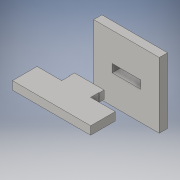
# Autodesk Inventor part: Part1
Saved by Autodesk Inventor 2016 (Build 200138000, 138)
## iProperties
Created: 2017-09-21
Part Number: Part1
Material: Generic
Document SubType Name: Modeling
Designer: student
Density: 1 g/cm^3
Appearance: Default
Author: student
Autodesk Inventor part; units mm, degrees
ref_plane "YZ Plane" through (0, 0, 0) normal (1, 0, 0) x (0, 1, 0)
ref_plane "XZ Plane" through (0, 0, 0) normal (0, 1, 0) x (-1, 0, 0)
ref_plane "XY Plane" through (0, 0, 0) normal (0, 0, 1) x (1, 0, 0)
sketch "Sketch1" plane through (0, 0, 0) normal (0, 0, 1) x (1, 0, 0)
  line L0 (-14.792, -1.3102) -> (-14.792, 1.814)
  line L1 (-14.792, 1.814) -> (-3.743, 1.814)
  line L2 (-3.743, 1.814) -> (-3.743, -1.3102)
  line L3 (-3.743, -1.3102) -> (-14.792, -1.3102)
  line L4 (-21.9675, -12.4544) -> (3.4325, -12.4544)
  line L5 (3.4325, -12.4544) -> (3.4325, 12.9456)
  line L6 (3.4325, 12.9456) -> (-21.9675, 12.9456)
  line L7 (-21.9675, 12.9456) -> (-21.9675, -12.4544)
  line L8 (-21.9675, -12.4544) -> (3.4325, 12.9456) construction
  line L9 (3.4325, -12.4544) -> (-21.9675, 12.9456) construction
  point P0 (0, 0)
  point P1 (-9.2675, 0.2456)
  dimension "d0" = 3.1242
  dimension "d2" = 11.049
  dimension "d3" = 25.4
  dimension "d4" = 25.4
  constraints: 20 end point, 2 horizontal, 2 midpoint, 2 parallel, 2 perpendicular, 2 vertical
  measures "d0" distance of L0.start L0.end
  measures "d2" distance of L0.end L1.end
  measures "d3" distance of L6.end L5.end
  measures "d4" distance of L5.end L4.end
extrude "Extrusion1" add sketch "Sketch1" along normal blind 3.175
sketch "Sketch2" plane through (0, 0, 0) normal (0, 1, 0) x (-1, 0, 0)
  line L0 (17.4601, 16.8923) -> (17.4601, 20.0673)
  line L1 (6.2587, 16.8923) -> (6.2587, 20.0673)
  line L2 (6.2587, 20.0673) -> (-3.2663, 20.0673)
  line L3 (17.4601, 20.0673) -> (26.9851, 20.0673)
  line L4 (26.9851, 20.0673) -> (26.9851, 29.5923)
  line L5 (26.9851, 29.5923) -> (-3.2663, 29.5923)
  line L6 (-3.2663, 29.5923) -> (-3.2663, 20.0673)
  line L7 (17.4601, 16.8923) -> (17.5871, 16.8923)
  line L8 (6.2587, 16.8923) -> (6.1317, 16.8923)
  line L9 (6.1317, 16.8923) -> (6.1317, 14.9873)
  line L10 (6.1317, 14.9873) -> (17.5871, 14.9873)
  line L11 (17.5871, 14.9873) -> (17.5871, 16.8923)
  point P0 (0, 0)
  dimension "d10" = 9.525
  dimension "d11" = 9.525
  dimension "d12" = 9.525
  dimension "d14" = 0.127
  dimension "d15" = 0.127
  dimension "d16" = 1.905
  dimension "d19" = 11.2014
  dimension "d20" = 11.4554
  constraints: 24 end point, 5 horizontal, 4 vertical, 2 perpendicular, 1 parallel
  measures "d10" distance of L1.end L2.end
  measures "d11" distance of L0.end L3.end
  measures "d12" distance of L3.end L4.end
  measures "d14" distance of L0.start L7.end
  measures "d15" distance of L1.start L8.end
  measures "d16" distance of L8.end L9.end
  measures "d19" distance between parallel lines of L1 L0
  measures "d20" distance between parallel lines of L9 L11
extrude "Extrusion2" add sketch "Sketch2" along normal blind 3.175
body "Solid1"
